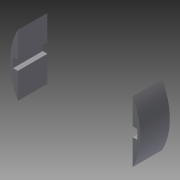
# Autodesk Inventor part: TRZYMACZ PCB
Saved by Autodesk Inventor 2014 (Build 180170000, 170)
## iProperties
Created: 2017-04-13
Part Number: TRZYMACZ PCB
Material: Ogólny
Document SubType Name: Modeling
Designer: hpdc7700
Density: 1 g/cm^3
Appearance: Domyślna
Author: hpdc7700
Autodesk Inventor part; units mm, degrees
ref_plane "YZ Plane" through (0, 0, 0) normal (1, 0, 0) x (0, 1, 0)
ref_plane "XZ Plane" through (0, 0, 0) normal (0, 1, 0) x (-1, 0, 0)
ref_plane "XY Plane" through (0, 0, 0) normal (0, 0, 1) x (1, 0, 0)
sketch "Szkic1" plane through (0, 0, 0) normal (0, 1, 0) x (-1, 0, 0)
  line L0 (-10.5, -0.8) -> (-8.9, -0.8)
  line L1 (-9.7, 0.8) -> (-10.5, 0.8)
  line L2 (-10.5, 0.8) -> (-10.5, -0.8)
  line L3 (-10.5, -0.8) -> (-8.9, 0.8) construction
  line L4 (-8.9, -0.8) -> (-10.5, 0.8) construction
  line L5 (9.7, 0.8) -> (10.5, 0.8)
  line L6 (10.5, 0.8) -> (10.5, -0.8)
  line L7 (10.5, -0.8) -> (9.7, -0.8)
  line L8 (8.9, 0.8) -> (10.5, -0.8) construction
  line L9 (10.5, 0.8) -> (8.9, -0.8) construction
  arc A0 (-9.7, 5.1875) -> (-9.7, -5.1875) centre (0, 0) ccw
  arc A1 (-5.7952, -9.3496) -> (5.7952, -9.3496) centre (0, 0) ccw
  arc A2 (9.7, -5.1875) -> (9.7, 5.1875) centre (0, 0) ccw
  line L10 (-9.7, -5.1875) -> (-9.7, -0.8)
  line L11 (-9.7, 0.8) -> (-9.7, 5.1875)
  line L12 (9.7, 5.1875) -> (9.7, 0.8)
  line L13 (9.7, -0.8) -> (9.7, -5.1875)
  point P0 (-9.7, 0)
  point P1 (9.7, 0)
  dimension "d5" = 21
  constraints: 28 end point, 6 parallel, 6 point on circle, 5 midpoint, 3 centre point, 2 horizontal, 1 coincident, 1 perpendicular
  measures "d5" distance between parallel lines of L6 L2
extrude "Wyciągnięcie proste1" add sketch "Szkic1" along normal blind 5
